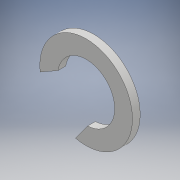
# Autodesk Inventor part: RetainingRingSmall
Saved by Autodesk Inventor 2018 (Build 220112000, 112)
## iProperties
Created: 2017-06-02
Part Number: RetainingRingSmall
Material: Generic
Document SubType Name: Modeling
Designer: Damian
Density: 1 g/cm^3
Appearance: Default
Author: Damian
Autodesk Inventor part; units mm, degrees
ref_plane "YZ Plane" through (0, 0, 0) normal (1, 0, 0) x (0, 1, 0)
ref_plane "XZ Plane" through (0, 0, 0) normal (0, 1, 0) x (-1, 0, 0)
ref_plane "XY Plane" through (0, 0, 0) normal (0, 0, 1) x (1, 0, 0)
sketch "Sketch1" plane through (0, 0, 0) normal (0, 1, 0) x (-1, 0, 0)
  arc A0 (1.9199, 2.1523) -> (0, 0) centre (0.0952, 1.8476) ccw
  arc A1 (3.0741, 1.4926) -> (0.7867, -1.0716) centre (0.0952, 1.8476) ccw
  line L0 (0, 0) -> (0.7867, -1.0716)
  line L1 (1.9199, 2.1523) -> (3.0741, 1.4926)
  dimension "d0" = 1.85
  dimension "d1" = 3
  dimension "d2" = 0
  dimension "d3" = 0
  constraints: 4 end point, 4 point on circle, 2 centre point, 1 equal length
  measures "d0" radius of A0
  measures "d1" radius of A1
  measures "d2" distance of A0.centre A1.centre
  measures "d3" distance of A1.centre A0.centre
extrude "Extrusion1" add sketch "Sketch1" along normal blind 0.5
body "Solid1"
